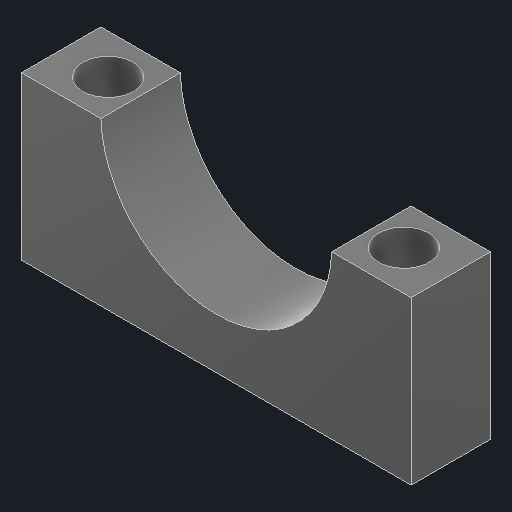
# Autodesk Inventor part: 16mm_Tube_Connecotor_Holybro
Saved by Autodesk Inventor 2025 (Build 290162010, 162A)
## iProperties
Created: 2023-06-08
Part Number: 16mm_Tube_Connecotor_Holybro
Material: ABS Plastic
Document SubType Name: Modeling
Designer: dzw04
Density: 1.06 g/cm^3
Appearance: Smooth - Black
Author: dzw04
Autodesk Inventor part; units mm, degrees
ref_plane "YZ Plane" through (0, 0, 0) normal (1, 0, 0) x (0, 1, 0)
ref_plane "XZ Plane" through (0, 0, 0) normal (0, 1, 0) x (-1, 0, 0)
ref_plane "XY Plane" through (0, 0, 0) normal (0, 0, 1) x (1, 0, 0)
sketch "Sketch1" plane through (0, 0, 0) normal (0, 0, 1) x (1, 0, 0)
  circle A0 centre (0, 0) radius 8
  line L0 (-13.5, -11.5) -> (13.5, -11.5)
  line L1 (13.5, -11.5) -> (13.5, 11.5)
  line L2 (13.5, 11.5) -> (-13.5, 11.5)
  line L3 (-13.5, 11.5) -> (-13.5, -11.5)
  line L4 (-13.5, -11.5) -> (13.5, 11.5) construction
  line L5 (13.5, -11.5) -> (-13.5, 11.5) construction
  line L6 (-13.5, -0.25) -> (13.5, -0.25)
  point P0 (7.9961, -0.25)
  point P1 (-7.9961, -0.25)
  dimension "d0" = 16
  dimension "d1" = 27
  dimension "d2" = 23
  dimension "d3" = 11.25
  constraints: 14 end point, 2 midpoint, 2 parallel, 2 perpendicular, 2 point on line, 1 centre point, 1 coincident, 1 horizontal
  measures "d0" diameter of A0
  measures "d1" distance of L2.end L1.end
  measures "d2" distance of L1.end L0.end
  measures "d3" distance between parallel lines of L0 L6
extrude "Extrusion1" add sketch "Sketch1" along normal blind 5.5 contours A0 L6 L1 L0 L3
sketch "Sketch2" plane through (-13.5, -11.5, 0) normal (0, -1, 0) x (1, 0, 0)
  line L0 (0, 0) -> (0, 5.5) projected
  line L1 (0, 2.75) -> (27, 2.75) construction
  line L2 (27, 0) -> (27, 5.5) projected
  circle A0 centre (23.75, 2.75) radius 1.75
  circle A1 centre (3.25, 2.75) radius 1.75
  point P0 (13.5, 0)
  point P1 (13.5, 2.75)
  dimension "d6" = 3.5
  dimension "d7" = 3.5
  dimension "d8" = 10.25
  dimension "d9" = 10.25
  constraints: 3 midpoint, 2 centre point, 2 end point, 2 point on line
  measures "d6" diameter of A0
  measures "d7" diameter of A1
  measures "d8" distance of A0.centre point (13.5, 2.75)
  measures "d9" distance of A1.centre point (13.5, 2.75)
extrude "Extrusion2" cut sketch "Sketch2" against normal through all
body "Solid1"
